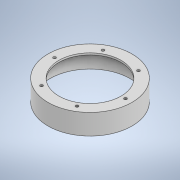
# Autodesk Inventor part: Diffuser_Top_Cover
Saved by Autodesk Inventor 2020 (Build 240168000, 168)
## iProperties
Created: 2021-04-25
Part Number: Diffuser_Top_Cover
Material: Generic
Document SubType Name: Modeling
Designer: Workshop
Density: 1 g/cm^3
Appearance: Default
Author: Workshop
Autodesk Inventor part; units mm, degrees
ref_plane "YZ Plane" through (0, 0, 0) normal (1, 0, 0) x (0, 1, 0)
ref_plane "XZ Plane" through (0, 0, 0) normal (0, 1, 0) x (-1, 0, 0)
ref_plane "XY Plane" through (0, 0, 0) normal (0, 0, 1) x (1, 0, 0)
sketch "Sketch1" plane through (0, 0, 0) normal (0, 0, 1) x (1, 0, 0)
  line L0 (0, 34.15) -> (-2, 34.15)
  line L1 (-2, 34.15) -> (-2, 46.15)
  line L2 (-2, 46.15) -> (20.5, 46.15)
  line L3 (20.5, 46.15) -> (20.5, 44.15)
  line L4 (20.5, 44.15) -> (0, 44.15)
  line L5 (0, 44.15) -> (0, 34.15)
  line L6 (-6.5, 0) -> (25, 0) projected
  point P0 (0, 0)
  dimension "d0" = 22.5
  dimension "d1" = 12
  dimension "d2" = 2
  dimension "d3" = 44.15
  dimension "d4" = 2
  constraints: 12 end point, 5 perpendicular, 1 horizontal, 1 vertical alignment
  measures "d0" distance of L1.end L2.end
  measures "d1" distance of L0.end L1.end
  measures "d2" distance of L2.end L3.end
  measures "d3" distance from line of point (0, 0) L4
  measures "d4" distance of L0.start L0.end
revolve "Revolution1" add sketch "Sketch1" angle 360 about axis through (-10, 0, 0) along (1, 0, 0)
sketch "Sketch2" plane through (-2, 0, 0) normal (-1, 0, 0) x (0, 0, 1)
  circle A0 centre (0, 39) radius 1.5
  point P0 (0, 0)
  dimension "d6" = 3
  dimension "d7" = 39
  constraints: 1 centre point, 1 vertical alignment
  measures "d6" diameter of A0
  measures "d7" distance of point (0, 0) A0.centre
extrude "Extrusion1" cut sketch "Sketch2" against normal through all
pattern_circular "Circular Pattern1" count 6 over 360 about axis through (9.25, 0, 0) along (1, 0, 0) of "Extrusion1"
body "Solid1"
